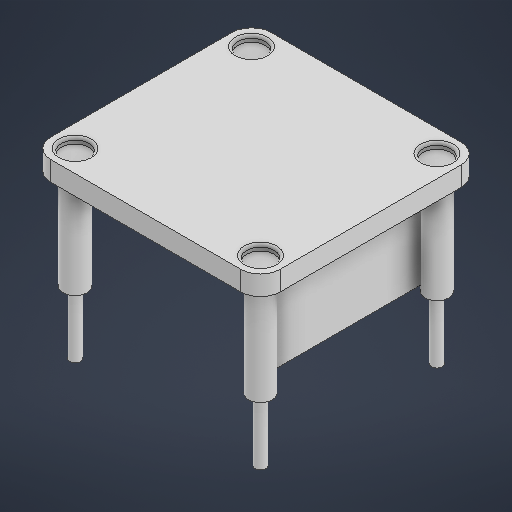
# Autodesk Inventor part: NUCCover_wall
Saved by Autodesk Inventor 2026 (Build 300175050, 175E)
## iProperties
Created: 2025-05-11
Part Number: NUCCover_wall
Material: Generic
Document SubType Name: Modeling
Designer: Sachi
Density: 1 g/cm^3
Appearance: Default
Author: Sachi
Autodesk Inventor part; units mm, degrees
ref_plane "YZ Plane" through (0, 0, 0) normal (1, 0, 0) x (0, 1, 0)
ref_plane "XZ Plane" through (0, 0, 0) normal (0, 1, 0) x (-1, 0, 0)
ref_plane "XY Plane" through (0, 0, 0) normal (0, 0, 1) x (1, 0, 0)
sketch "Sketch1" plane through (0, 0, 0) normal (0, 1, 0) x (-1, 0, 0)
  circle A0 centre (-2.7724, -39.7021) radius 1.9558
  circle A1 centre (-2.7724, 44.6259) radius 1.9558
  circle A2 centre (-50.0164, -42.4961) radius 6.0325
  circle A3 centre (44.4716, 47.4199) radius 6.0325
  circle A4 centre (44.4716, -42.4961) radius 6.0325
  circle A5 centre (-50.0164, 47.4199) radius 6.0325
  line L0 (-61.1924, -53.6721) -> (55.6476, -53.6721)
  line L1 (55.6476, -53.6721) -> (55.6476, 58.5959)
  line L2 (55.6476, 58.5959) -> (-61.1924, 58.5959)
  line L3 (-61.1924, 58.5959) -> (-61.1924, -53.6721)
  line L4 (36.8516, 55.4209) -> (36.8516, 39.7999)
  line L5 (36.8516, 39.7999) -> (52.4726, 39.7999)
  line L6 (52.4726, 39.7999) -> (52.4726, -34.8761)
  line L7 (52.4726, -34.8761) -> (36.8516, -34.8761)
  line L8 (36.8516, -34.8761) -> (36.8516, -50.4971)
  line L9 (-42.3964, -50.4971) -> (-42.3964, -34.8761)
  line L10 (-42.3964, -34.8761) -> (-58.0174, -34.8761)
  line L11 (-58.0174, -34.8761) -> (-58.0174, 39.7999)
  line L12 (-58.0174, 39.7999) -> (-42.3964, 39.7999)
  line L13 (-42.3964, 39.7999) -> (-42.3964, 55.4209)
  line L14 (-42.3964, -50.4971) -> (-7.8524, -50.4971)
  line L15 (-7.8524, -50.4971) -> (-7.8524, -34.8761)
  line L16 (-7.8524, -34.8761) -> (2.3076, -34.8761)
  line L17 (2.3076, -34.8761) -> (2.3076, -50.4971)
  line L18 (2.3076, -50.4971) -> (36.8516, -50.4971)
  line L19 (-42.3964, 55.4209) -> (-7.8524, 55.4209)
  line L20 (-7.8524, 55.4209) -> (-7.8524, 39.7999)
  line L21 (-7.8524, 39.7999) -> (2.3076, 39.7999)
  line L22 (2.3076, 39.7999) -> (2.3076, 55.4209)
  line L23 (2.3076, 55.4209) -> (36.8516, 55.4209)
  circle A6 centre (-50.0164, 47.4199) radius 2.75
  circle A7 centre (-50.0164, -42.4961) radius 2.75
  circle A8 centre (44.4716, 47.4199) radius 2.75
  circle A9 centre (44.4716, -42.4961) radius 2.75
  point P0 (0, 0)
  point P1 (-2.7724, 2.4619)
  dimension "d0" = 3.175
  dimension "d1" = 15.621
  dimension "d2" = 15.621
  dimension "d3" = 15.621
  dimension "d4" = 3.175
  dimension "d5" = 5.08
  dimension "d6" = 5.08
  dimension "d7" = 3.175
  dimension "d8" = 3.175
  dimension "d22" = 5.5
  dimension "d23" = 5.5
  dimension "d24" = 5.5
  dimension "d25" = 5.5
  constraints: 48 end point, 15 perpendicular, 10 centre point, 7 equal length, 4 coincident, 3 point on line, 2 horizontal, 1 collinear, 1 vertical
  measures "d0" distance between parallel lines of L3 L11
  measures "d1" distance of L12.end L13.end
  measures "d2" distance of L7.end L8.end
  measures "d3" distance of L9.end L10.end
  measures "d4" distance between parallel lines of L1 L6
  measures "d5" distance from line of A0.centre L17
  measures "d6" distance from line of A0.centre L15
  measures "d7" distance between parallel lines of L0 L14
  measures "d8" distance between parallel lines of L2 L19
  measures "d22" diameter of A8
  measures "d23" diameter of A9
  measures "d24" diameter of A7
  measures "d25" diameter of A6
extrude "Extrusion1" add sketch "Sketch1" along normal blind 50.8 contours A2 | A3 | A4 | A5 | A6 | A7 | A8 | A9
extrude "Extrusion2" add sketch "Sketch1" along normal blind 10 from surface at 50.8 contours A0 | A1 | A2 | A3 | A4 | A5 | L3 L2 L1 L0 | L4 L5 L6 L7 L8 L18 L17 L16 L15 L14 L9 L10 L11 L12 L13 L19 L20 L21 L22 L23 | A6 | A7 | A8 | A9
fillet "Fillet1" radius 10 4 edges at (61.1924, 55.8, 58.5959) (-55.6476, 55.8, 58.5959) (-55.6476, 55.8, -53.6721) (61.1924, 55.8, -53.6721)
extrude "Extrusion3" add sketch "Sketch1" against normal blind 32 contours A6 | A7 | A8 | A9
sketch "Sketch4" plane through (-45.6476, 50.8, 58.5959) normal (0, -1, 0) x (1, 0, 0)
  circle A0 centre (95.664, -11.176) radius 6.0325 projected
  circle A1 centre (95.664, -101.092) radius 6.0325 projected
  line L0 (89.6315, -11.176) -> (89.6315, -101.092)
  line L1 (89.6315, -101.092) -> (88.6315, -101.092)
  line L2 (88.6315, -101.092) -> (88.6315, -11.176)
  line L3 (88.6315, -11.176) -> (89.6315, -11.176)
  point P0 (45.6476, -58.5959)
  dimension "d46" = 1
  constraints: 8 end point, 2 horizontal alignment, 2 parallel, 1 perpendicular, 1 vertical, 2 other
  measures "d46" distance of L2.end L0.start
extrude "Extrusion4" add sketch "Sketch4" along normal blind 50 contours L0 L1 L2 L3
sketch "Sketch6" plane through (-45.6476, 60.8, -53.6721) normal (0, 1, 0) x (1, 0, 0)
  circle A0 centre (1.176, -11.176) radius 7
  line L0 (0, 0) -> (96.84, 0) projected
  line L1 (0, 0) -> (96.84, 0)
  line L2 (-10, -102.268) -> (-10, -10) projected
  line L3 (-10, -10) -> (-10, -102.268)
  arc A1 (96.84, -112.268) -> (106.84, -102.268) centre (96.84, -102.268) ccw projected
  line L4 (0, -112.268) -> (96.84, -112.268)
  line L5 (106.84, -10) -> (106.84, -102.268) projected
  line L6 (106.84, -102.268) -> (106.84, -10)
  circle A2 centre (95.664, -11.176) radius 7
  circle A3 centre (1.176, -101.092) radius 7
  circle A4 centre (95.664, -101.092) radius 7
  arc A5 (0, 0) -> (-10, -10) centre (0, -10) ccw
  arc A6 (-10, -102.268) -> (0, -112.268) centre (0, -102.268) ccw projected
  arc A7 (-10, -102.268) -> (0, -112.268) centre (0, -102.268) ccw
  arc A8 (106.84, -10) -> (96.84, 0) centre (96.84, -10) ccw
  point P0 (45.6476, -53.6721)
  dimension "d30" = 14
  dimension "d33" = 14
  dimension "d36" = 11.176
  dimension "d38" = 11.176
  dimension "d39" = 11.176
  dimension "d40" = 11.176
  dimension "d43" = 14
  dimension "d44" = 14
  dimension "d47" = 11.176
  dimension "d48" = 11.176
  dimension "d49" = 11.176
  dimension "d51" = 11.176
  constraints: 8 end point, 7 centre point, 6 point on circle, 4 tangent, 2 collinear, 1 horizontal, 1 vertical
  measures "d30" diameter of A0
  measures "d33" diameter of A2
  measures "d36" distance from line of L5 A2.centre
  measures "d38" vertical distance of L4.start A3.centre
  measures "d39" distance from line of L4 A4.centre
  measures "d40" distance from line of L6 A4.centre
  measures "d43" diameter of A3
  measures "d44" diameter of A4
  measures "d47" horizontal distance of L2.end A0.centre
  measures "d48" vertical distance of L0.start A0.centre
  measures "d49" vertical distance of L0.end A2.centre
  measures "d51" distance from line of L3 A3.centre
extrude "Extrusion5" cut sketch "Sketch6" against normal blind 3 contours A0 | A2 | A3 | A4
fillet "Fillet2" radius 1.3 4 edges at (43.0164, 60.8, 47.4199) (-51.4716, 60.8, 47.4199) (-51.4716, 60.8, -42.4961) (43.0164, 60.8, -42.4961)
equation "\"d2\" = d1"
equation "\"d3\" = d1"
equation "\"d4\" = d0"
equation "\"d6\" = d5"
equation "\"d7\" = d0"
equation "\"d8\" = d0"
body "Solid1"
